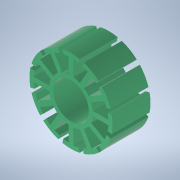
# Autodesk Inventor part: STATOR
Saved by Autodesk Inventor 2022 (Build 260153000, 153)
## iProperties
Created: 2022-07-26
Part Number: STATOR
Material: Generic
Document SubType Name: Modeling
Designer: Nathan Cai
Density: 1 g/cm^3
Appearance: Rubber - Green
Author: Nathan Cai
Autodesk Inventor part; units mm, degrees
ref_plane "YZ Plane" through (0, 0, 0) normal (1, 0, 0) x (0, 1, 0)
ref_plane "XZ Plane" through (0, 0, 0) normal (0, 1, 0) x (-1, 0, 0)
ref_plane "XY Plane" through (0, 0, 0) normal (0, 0, 1) x (1, 0, 0)
sketch "Sketch1" plane through (0, 0, 0) normal (0, 0, 1) x (1, 0, 0)
  arc A0 (-17.1176, 3.6385) -> (-17.1176, -3.6385) centre (0, 0) ccw
  circle A1 centre (0, 0) radius 7.5
  arc A2 (-15.4058, 3.2746) -> (-15.4058, -3.2746) centre (0, 0) ccw
  circle A3 centre (0, 0) radius 9.25
  line L0 (0, 0) -> (-17.5, 0) construction
  line L1 (-15.7182, -1) -> (-9.1958, -1)
  line L2 (-15.7182, 1) -> (-9.1958, 1)
  line L3 (-15.4058, 3.2746) -> (-17.1176, 3.6385)
  line L4 (-15.4058, -3.2746) -> (-17.1176, -3.6385)
  line L5 (0, 0) -> (-17.1176, 3.6385) construction
  arc A4 (-16.6435, -5.4078) -> (-13.005, -11.7098) centre (0, 0) ccw
  arc A5 (-14.9791, -4.867) -> (-11.7045, -10.5388) centre (0, 0) ccw
  line L6 (-13.1124, -8.7251) -> (-7.4638, -5.4639)
  line L7 (-14.1124, -6.9931) -> (-8.4638, -3.7319)
  line L8 (-14.9791, -4.867) -> (-16.6435, -5.4078)
  line L9 (-11.7045, -10.5388) -> (-13.005, -11.7098)
  arc A6 (-11.7098, -13.005) -> (-5.4078, -16.6435) centre (0, 0) ccw
  arc A7 (-10.5388, -11.7045) -> (-4.867, -14.9791) centre (0, 0) ccw
  line L10 (-6.9931, -14.1124) -> (-3.7319, -8.4638)
  line L11 (-8.7251, -13.1124) -> (-5.4639, -7.4638)
  line L12 (-10.5388, -11.7045) -> (-11.7098, -13.005)
  line L13 (-4.867, -14.9791) -> (-5.4078, -16.6435)
  arc A8 (-3.6385, -17.1176) -> (3.6385, -17.1176) centre (0, 0) ccw
  arc A9 (-3.2746, -15.4058) -> (3.2746, -15.4058) centre (0, 0) ccw
  line L14 (1, -15.7182) -> (1, -9.1958)
  line L15 (-1, -15.7182) -> (-1, -9.1958)
  line L16 (-3.2746, -15.4058) -> (-3.6385, -17.1176)
  line L17 (3.2746, -15.4058) -> (3.6385, -17.1176)
  arc A10 (5.4078, -16.6435) -> (11.7098, -13.005) centre (0, 0) ccw
  arc A11 (4.867, -14.9791) -> (10.5388, -11.7045) centre (0, 0) ccw
  line L18 (8.7251, -13.1124) -> (5.4639, -7.4638)
  line L19 (6.9931, -14.1124) -> (3.7319, -8.4638)
  line L20 (4.867, -14.9791) -> (5.4078, -16.6435)
  line L21 (10.5388, -11.7045) -> (11.7098, -13.005)
  arc A12 (13.005, -11.7098) -> (16.6435, -5.4078) centre (0, 0) ccw
  arc A13 (11.7045, -10.5388) -> (14.9791, -4.867) centre (0, 0) ccw
  line L22 (14.1124, -6.9931) -> (8.4638, -3.7319)
  line L23 (13.1124, -8.7251) -> (7.4638, -5.4639)
  line L24 (11.7045, -10.5388) -> (13.005, -11.7098)
  line L25 (14.9791, -4.867) -> (16.6435, -5.4078)
  arc A14 (17.1176, -3.6385) -> (17.1176, 3.6385) centre (0, 0) ccw
  arc A15 (15.4058, -3.2746) -> (15.4058, 3.2746) centre (0, 0) ccw
  line L26 (15.7182, 1) -> (9.1958, 1)
  line L27 (15.7182, -1) -> (9.1958, -1)
  line L28 (15.4058, -3.2746) -> (17.1176, -3.6385)
  line L29 (15.4058, 3.2746) -> (17.1176, 3.6385)
  arc A16 (16.6435, 5.4078) -> (13.005, 11.7098) centre (0, 0) ccw
  arc A17 (14.9791, 4.867) -> (11.7045, 10.5388) centre (0, 0) ccw
  line L30 (13.1124, 8.7251) -> (7.4638, 5.4639)
  line L31 (14.1124, 6.9931) -> (8.4638, 3.7319)
  line L32 (14.9791, 4.867) -> (16.6435, 5.4078)
  line L33 (11.7045, 10.5388) -> (13.005, 11.7098)
  arc A18 (11.7098, 13.005) -> (5.4078, 16.6435) centre (0, 0) ccw
  arc A19 (10.5388, 11.7045) -> (4.867, 14.9791) centre (0, 0) ccw
  line L34 (6.9931, 14.1124) -> (3.7319, 8.4638)
  line L35 (8.7251, 13.1124) -> (5.4639, 7.4638)
  line L36 (10.5388, 11.7045) -> (11.7098, 13.005)
  line L37 (4.867, 14.9791) -> (5.4078, 16.6435)
  arc A20 (3.6385, 17.1176) -> (-3.6385, 17.1176) centre (0, 0) ccw
  arc A21 (3.2746, 15.4058) -> (-3.2746, 15.4058) centre (0, 0) ccw
  line L38 (-1, 15.7182) -> (-1, 9.1958)
  line L39 (1, 15.7182) -> (1, 9.1958)
  line L40 (3.2746, 15.4058) -> (3.6385, 17.1176)
  line L41 (-3.2746, 15.4058) -> (-3.6385, 17.1176)
  arc A22 (-5.4078, 16.6435) -> (-11.7098, 13.005) centre (0, 0) ccw
  arc A23 (-4.867, 14.9791) -> (-10.5388, 11.7045) centre (0, 0) ccw
  line L42 (-8.7251, 13.1124) -> (-5.4639, 7.4638)
  line L43 (-6.9931, 14.1124) -> (-3.7319, 8.4638)
  line L44 (-4.867, 14.9791) -> (-5.4078, 16.6435)
  line L45 (-10.5388, 11.7045) -> (-11.7098, 13.005)
  arc A24 (-13.005, 11.7098) -> (-16.6435, 5.4078) centre (0, 0) ccw
  arc A25 (-11.7045, 10.5388) -> (-14.9791, 4.867) centre (0, 0) ccw
  line L46 (-14.1124, 6.9931) -> (-8.4638, 3.7319)
  line L47 (-13.1124, 8.7251) -> (-7.4638, 5.4639)
  line L48 (-11.7045, 10.5388) -> (-13.005, 11.7098)
  line L49 (-14.9791, 4.867) -> (-16.6435, 5.4078)
  point P0 (-15.1554, -8.75)
  point P1 (-8.75, -15.1554)
  point P2 (0, -17.5)
  point P3 (8.75, -15.1554)
  point P4 (15.1554, -8.75)
  point P5 (17.5, 0)
  point P6 (15.1554, 8.75)
  point P7 (8.75, 15.1554)
  point P8 (0, 17.5)
  point P9 (-8.75, 15.1554)
  point P10 (-15.1554, 8.75)
  dimension "d0" = 35
  dimension "d1" = 15
  dimension "d2" = 1.75
  dimension "d3" = 1.75
  dimension "d6" = 1
  dimension "d7" = 12
  dimension "d10" = 360
  constraints: 100 end point, 84 point on circle, 25 centre point, 2 coincident, 2 symmetric about line, 1 collinear, 1 horizontal, 1 parallel, 197 other
  measures "d0" diameter of A0
  measures "d1" diameter of A1
  measures "d2" radial gap between concentric circles of A0 A2
  measures "d6" distance between parallel lines of L0 L2
  measures "d7" angle of L0 L3
extrude "Extrusion1" add sketch "Sketch1" along normal blind 16
body "Solid1"
